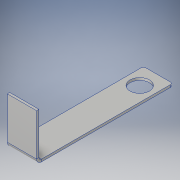
# Autodesk Inventor part: Soporte - Ruedas Delanteras
Saved by Autodesk Inventor 2019 (Build 230136000, 136)
## iProperties
Created: 2019-11-14
Part Number: Soporte - Ruedas Delanteras
Material: Aluminio 6061
Document SubType Name: Chapa
Designer: eddysanoli
Density: 2.7 g/cm^3
Sheet Metal Rule: Por defecto_mm
Appearance: Aluminio - Plano
Mass: 4.61307 g
Surface Area: 70.2464 cm^2
Volume: 1.70854 cm^3
Author: eddysanoli
Autodesk Inventor part; units mm, degrees
ref_plane "YZ Plane" through (0, 0, 0) normal (1, 0, 0) x (0, 1, 0)
ref_plane "XZ Plane" through (0, 0, 0) normal (0, 1, 0) x (-1, 0, 0)
ref_plane "XY Plane" through (0, 0, 0) normal (0, 0, 1) x (1, 0, 0)
sketch "Boceto1" plane through (0, 0, 0) normal (0, 1, 0) x (-1, 0, 0)
  line L0 (0, 0) -> (23.85, 0)
  line L1 (23.85, 0) -> (23.85, -107.5)
  line L2 (21.85, -109.5) -> (2, -109.5)
  line L3 (0, -107.5) -> (0, 0)
  line L4 (0, 0) -> (23.85, 0)
  line L5 (23.85, 0) -> (23.85, 36.5)
  line L6 (23.85, 36.5) -> (0, 36.5)
  line L7 (0, 36.5) -> (0, 0)
  circle A0 centre (11.925, -94.5) radius 7.95
  arc A1 (21.85, -109.5) -> (23.85, -107.5) centre (21.85, -107.5) ccw
  arc A2 (0, -107.5) -> (2, -109.5) centre (2, -107.5) ccw
  point P0 (23.85, -109.5)
  point P1 (0, -109.5)
  point P2 (11.925, 36.5)
  dimension "d0" = 94.5
  dimension "d1" = 15
  dimension "d2" = 15.9
  dimension "d3" = 23.85
  dimension "d4" = 36.5
  dimension "d12" = 2
  constraints: 16 end point, 5 point on line, 4 parallel, 4 point on circle, 4 tangent, 3 centre point, 2 horizontal, 2 perpendicular, 1 equal radius, 1 midpoint, 1 vertical alignment
  measures "d0" distance from line of A0.centre L0
  measures "d1" distance from line of L2 A0.centre
  measures "d2" diameter of A0
  measures "d3" distance between parallel lines of L5 L7
  measures "d4" distance between parallel lines of L0 L6
  measures "d12" radius of A1
extrude "Placa1" add sketch "Boceto1" along normal blind 2
fold "Pliegue1" angle 90 bend radius 2 thickness 2 k factor 0.44 line from (0, 0, 0) to (-23.85, 0, 0) line at bend centre moving side (0, 0, 1) folds toward (0, 1, 0)
equation "\"d3\" = 1.5 * d2"
equation "\"d4\" = 0.333333 * d1 + 0.333333 * d0"
equation "\"d5\" = Grosor"
equation "\"d6\" = Anchura_desahogo_plegado"
equation "\"d7\" = Profundidad_desahogo_plegado"
equation "\"d8\" = Remanente_mínimo"
equation "\"d9\" = Radiodetransición"
equation "\"d11\" = Radio_pliegue"
equation "\"Radio_pliegue\" = Grosor"
equation "\"Anchura_desahogo_plegado\" = Grosor"
equation "\"Profundidad_desahogo_plegado\" = 0.5 * Grosor"
equation "\"Tamaño_destalonado\" = 4 * Grosor"
equation "\"Remanente_mínimo\" = 2 * Grosor"
equation "\"Radiodetransición\" = Radio_pliegue"
equation "\"Tamaño_de_radio_de_Jacobi\" = Radio_pliegue"
equation "\"TamañoSeparación\" = Grosor"
equation "\"Grosor\" = 2"
